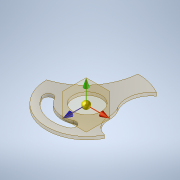
# Autodesk Inventor part: WeaponV1
Saved by Autodesk Inventor 2020 (Build 240168000, 168)
## iProperties
Created: 2023-11-25
Part Number: WeaponV1
Material: Titanium
Document SubType Name: Modeling
Designer: smz3rm
Mass: 36.6533 g
Surface Area: 68.2673 cm^2
Volume: 8.12711 cm^3
Density: 4.51 g/cm^3
Appearance: Titanium
Author: smz3rm
Autodesk Inventor part; units mm, degrees
ref_plane "YZ Plane" through (0, 0, 0) normal (1, 0, 0) x (0, 1, 0)
ref_plane "XZ Plane" through (0, 0, 0) normal (0, 1, 0) x (-1, 0, 0)
ref_plane "XY Plane" through (0, 0, 0) normal (0, 0, 1) x (1, 0, 0)
sketch "Sketch1" plane through (0, 0, 0) normal (0, 1, 0) x (-1, 0, 0)
  circle A0 centre (0, 0) radius 13.9
  circle A1 centre (0, 0) radius 50
  circle A2 centre (0, 0) radius 40
  arc A3 (40, 0) -> (0, -50) centre (57.7287, -55.183) ccw
  arc A4 (-25, -43.3013) -> (-40, 0) centre (-39.1119, -23.9411) ccw
  line L0 (0, -76.2196) -> (0, 71.0366) projected
  line L1 (79.2745, 0) -> (-71.5457, 0) projected
  circle A5 centre (0, 0) radius 21.9
  arc A6 (40, 0) -> (21.9, 0) centre (30.95, -10.4491) ccw
  arc A7 (-21.9, 0) -> (-35.49, 18.4516) centre (-39.9897, 0.907) ccw
  point P0 (1.8028, -39.9594)
  point P1 (-18.195, -35.6222)
  point P2 (0, -40)
  point P3 (-18.6785, -11.4334)
  point P4 (15.8308, -15.1326)
  dimension "d0" = 27.8
  dimension "d1" = 100
  dimension "d2" = 80
  dimension "d3" = 8
  dimension "d4" = 25
  dimension "d5" = 8
  constraints: 16 point on circle, 8 centre point, 5 point on line, 4 coincident, 1 tangent
  measures "d0" diameter of A0
  measures "d1" diameter of A1
  measures "d2" diameter of A2
  measures "d4" horizontal distance of A1.start A1.end
extrude "Extrusion1" add sketch "Sketch1" along normal blind 3 contours L1 A5 L0 A0 | A0 L0 A5 L1 | A0 L1 A7 A5 L0 | L0 A5 L1 A0 | A6 L1 | L1 A3 A5 | A5 L0 A2 A6 | A5 A7 A2 L0 | A5 A3 A2 L0 | L0 A2 A4 A5 | L0 A1 A4 A2 | A2 A3 L0
sketch "Sketch3" plane through (0, 3, 0) normal (0, 1, 0) x (1, 0, 0)
  arc A0 (-24.3734, -14.0416) -> (9.9475, -25.6733) centre (-1.1345, -1.9225) ccw construction
  arc A1 (-28.4861, -16.1864) -> (11.9088, -29.8767) centre (-1.1345, -1.9225) ccw
  arc A2 (-20.2606, -11.8967) -> (7.9863, -21.47) centre (-1.1345, -1.9225) ccw
  arc A3 (-20.2606, -11.8967) -> (-28.4861, -16.1864) centre (-24.3734, -14.0416) ccw
  arc A4 (11.9088, -29.8767) -> (7.9863, -21.47) centre (9.9475, -25.6733) ccw
  point P0 (0, 0)
  constraints: 10 point on circle, 5 centre point, 4 tangent
extrude "Extrusion3" cut sketch "Sketch3" against normal blind 3
body "Solid1"
